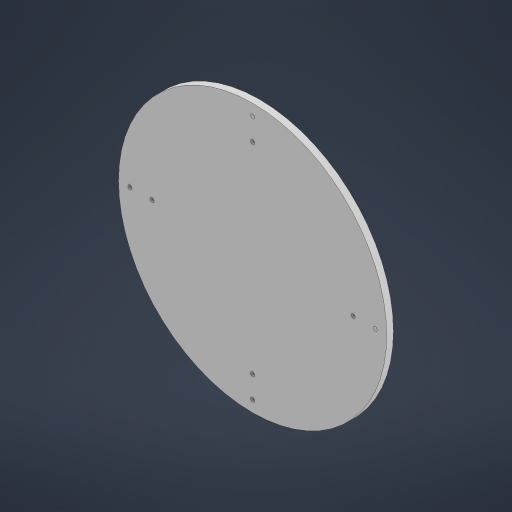
# Autodesk Inventor part: Components Base
Saved by Autodesk Inventor 2023 (Build 270158000, 158)
## iProperties
Created: 2023-04-06
Part Number: Components Base
Material: Generic
Document SubType Name: Modeling
Designer: vatdu
Density: 1 g/cm^3
Appearance: Default
Author: vatdu
Autodesk Inventor part; units mm, degrees
ref_plane "YZ Plane" through (0, 0, 0) normal (1, 0, 0) x (0, 1, 0)
ref_plane "XZ Plane" through (0, 0, 0) normal (0, 1, 0) x (-1, 0, 0)
ref_plane "XY Plane" through (0, 0, 0) normal (0, 0, 1) x (1, 0, 0)
sketch "Sketch1" plane through (0, 0, 0) normal (0, 0, 1) x (1, 0, 0)
  circle A0 centre (0, 0) radius 100
  circle A1 centre (0, 75) radius 1.5
  circle A2 centre (-75, 0) radius 1.5
  circle A3 centre (0, -75) radius 1.5
  circle A4 centre (75, 0) radius 1.5
  circle A5 centre (0, 91.5) radius 1.5
  circle A6 centre (91.5, 0) radius 1.5
  circle A7 centre (0, -91.5) radius 1.5
  circle A8 centre (-91.5, 0) radius 1.5
  dimension "d0" = 200
  dimension "d2" = 3
  dimension "d5" = 360
  dimension "d10" = 3
  dimension "d11" = 3
  dimension "d12" = 3
  dimension "d13" = 3
  constraints: 9 centre point, 1 coincident, 9 other
  measures "d0" diameter of A0
  measures "d2" diameter of A1
  measures "d10" diameter of A5
  measures "d11" diameter of A6
  measures "d12" diameter of A7
  measures "d13" diameter of A8
extrude "Extrusion1" add sketch "Sketch1" along normal blind 5
body "Solid1"
